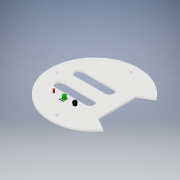
# Autodesk Inventor part: Top and middle round
Saved by Autodesk Inventor 2018 (Build 220112000, 112)
## iProperties
Created: 2018-10-22
Part Number: Top and middle round
Material: Generic
Document SubType Name: Modeling
Designer: Melda
Density: 1 g/cm^3
Appearance: White
Author: Melda
Autodesk Inventor part; units mm, degrees
ref_plane "YZ Plane" through (0, 0, 0) normal (1, 0, 0) x (0, 1, 0)
ref_plane "XZ Plane" through (0, 0, 0) normal (0, 1, 0) x (-1, 0, 0)
ref_plane "XY Plane" through (0, 0, 0) normal (0, 0, 1) x (1, 0, 0)
sketch "Sketch1" plane through (0, 0, 0) normal (0, 1, 0) x (-1, 0, 0)
  arc A0 (-99.8914, -75.1446) -> (-99.8914, 75.1446) centre (0, 0) ccw
  line L0 (-65, 0) -> (-65, 55)
  line L1 (-65, 55) -> (-99.8914, 75.1446)
  line L2 (-65, 0) -> (-65, -55)
  line L3 (-65, -55) -> (-99.8914, -75.1446)
  dimension "d0" = 250
  dimension "d4" = 55
  dimension "d6" = 120
  constraints: 8 end point, 2 point on circle, 1 centre point, 1 coincident, 1 vertical
  measures "d0" diameter of A0
  measures "d4" distance of L0.start L0.end
  measures "d6" angle of L1 L0
extrude "Extrusion1" add sketch "Sketch1" along normal blind 5
sketch "Sketch2" plane through (0, 5, 0) normal (0, 1, 0) x (1, 0, 0)
  line L0 (-70, 15) -> (15, 15)
  line L1 (15, 40) -> (-70, 40)
  arc A0 (15, 15) -> (15, 40) centre (15, 27.5) ccw
  arc A1 (-70, 40) -> (-70, 15) centre (-70, 27.5) ccw
  line L2 (65, -55) -> (65, 55) projected
  line L3 (-70, -15) -> (15, -15)
  line L4 (15, -40) -> (-70, -40)
  arc A2 (15, -40) -> (15, -15) centre (15, -27.5) ccw
  arc A3 (-70, -15) -> (-70, -40) centre (-70, -27.5) ccw
  point P0 (0, 0)
  constraints: 8 end point, 8 point on circle, 4 centre point, 2 tangent, 1 horizontal, 1 parallel
extrude "Extrusion2" cut sketch "Sketch2" against normal blind 10
sketch "Sketch3" plane through (0, 5, 0) normal (0, 1, 0) x (1, 0, 0)
  circle A0 centre (-105, 0) radius 4
  circle A1 centre (0, 105) radius 4.3333
  circle A2 centre (0, -105) radius 4.3461
  arc A3 (99.8914, 75.1446) -> (99.8914, -75.1446) centre (0, 0) ccw projected
  dimension "d25" = 8
  dimension "d26" = 105
  dimension "d27" = 105
  dimension "d28" = 105
  constraints: 3 centre point
  measures "d25" diameter of A0
  measures "d26" distance of A3.centre A0.centre
  measures "d27" distance of A3.centre A1.centre
  measures "d28" distance of A3.centre A2.centre
extrude "Extrusion3" cut sketch "Sketch3" against normal blind 10
sketch "Sketch4" plane through (0, 5, 0) normal (0, 1, 0) x (1, 0, 0)
  circle A0 centre (-59.9853, -55) radius 2.5
  circle A1 centre (-29.9853, -55) radius 5
  circle A2 centre (0.0147, -55) radius 5
  line L0 (-104.2134, 0) -> (86.9491, 0)
  point P0 (0, 0)
  dimension "d31" = 5
  dimension "d32" = 10
  dimension "d33" = 10
  dimension "d34" = 55
  dimension "d35" = 55
  dimension "d36" = 55
  dimension "d37" = 30
  dimension "d38" = 30
  constraints: 3 centre point, 2 end point, 1 horizontal
  measures "d31" diameter of A0
  measures "d32" diameter of A1
  measures "d33" diameter of A2
  measures "d34" distance from line of L0 A0.centre
  measures "d35" distance from line of L0 A1.centre
  measures "d36" distance from line of A2.centre L0
  measures "d37" distance of A1.centre A2.centre
  measures "d38" distance of A1.centre A0.centre
extrude "Extrusion4" add sketch "Sketch4" along normal blind 10
fillet "Fillet2" radius 2 1 edges at (-62.4853, 15, 55)
chamfer "Chamfer1" distance 1.25 angle 45 1 edges at (-4.9853, 15, 55)
chamfer "Chamfer2" distance 1.25 angle 45 1 edges at (-34.9853, 15, 55)
sketch "Sketch5" plane through (0, 5, 0) normal (0, 1, 0) x (1, 0, 0)
  line L0 (-35.937, -60.9099) -> (-23.937, -60.9099)
  line L1 (-23.937, -60.9099) -> (-23.937, -48.9099)
  line L2 (-23.937, -48.9099) -> (-35.937, -48.9099)
  line L3 (-35.937, -48.9099) -> (-35.937, -60.9099)
  point P0 (0, 0)
  point P1 (-29.437, -54.7059)
  point P2 (-29.437, -54.7059)
  dimension "d50" = 12
  dimension "d51" = 12
  dimension "d52" = 6.5
  dimension "d53" = 5.796
  constraints: 8 end point, 2 parallel, 1 coincident, 1 horizontal, 1 perpendicular
  measures "d50" distance between parallel lines of L1 L3
  measures "d51" distance between parallel lines of L0 L2
  measures "d52" distance from line of L3 point (-29.437, -54.706)
  measures "d53" distance from line of point (-29.437, -54.706) L2
extrude "Extrusion5" add sketch "Sketch5" along normal blind 0.05
sketch "Sketch6" plane through (0, 5, 0) normal (0, 1, 0) x (1, 0, 0)
  line L0 (-36.7143, -61.9407) -> (-23.1511, -61.9407) construction
  line L1 (-23.1511, -61.9407) -> (-23.1511, -65.2373) construction
  line L2 (-23.1511, -65.2373) -> (-36.7143, -65.2373) construction
  line L3 (-36.7143, -65.2373) -> (-36.7143, -61.9407) construction
  point P0 (0, 0)
  constraints: 2 other
body "Solid1"
